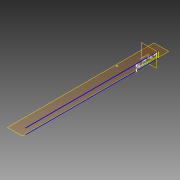
# Autodesk Inventor part: MotorHolder
Saved by Autodesk Inventor 2012 SP2 (Build 160219200, 219)
## iProperties
Created: 2014-02-06
Part Number: MotorHolder
Material: Default
Document SubType Name: Modeling
Designer: 1
Density: 1 g/cm^3
Author: 1
Autodesk Inventor part; units mm, degrees
ref_plane "YZ Plane" through (0, 0, 0) normal (1, 0, 0) x (0, 1, 0)
sketch "Sketch2" plane through (0, 0, 0) normal (1, 0, 0) x (0, 1, 0)
  line L0 (-26.7778, -143.959) -> (-26.7778, 317.1285)
  line L1 (-46.7778, -143.959) -> (-46.7778, 317.1285)
  line L2 (-26.7778, -143.959) -> (-46.7778, -143.959) projected
  line L3 (-39.365, -88.8667) -> (-41.365, -88.8667)
  line L4 (-41.365, -88.8667) -> (-41.365, -138.8667)
  line L5 (-41.365, -138.8667) -> (-39.365, -138.8667)
  line L6 (-39.365, -138.8667) -> (-39.365, -88.8667)
  point P0 (0, 0)
  dimension "d0" = 2
  dimension "d1" = 50
  constraints: 12 end point, 2 parallel, 2 vertical, 1 horizontal, 1 perpendicular, 4 other
  measures "d0" distance of L3.start L3.end
  measures "d1" distance of L3.end L4.end
ref_plane "Work Plane1" through (0, 0, -111.125) normal (0, 0, 1) x (1, 0, 0)
sketch "Sketch3" plane through (0, 0, -111.125) normal (0, 0, 1) x (1, 0, 0)
  line L0 (10, -547.5814) -> (10, 52.4186)
  circle A0 centre (-26.4569, -36.7778) radius 10 projected
  line L1 (-15.1483, -33.3426) -> (-15.1483, -63.4863)
  line L2 (-15.1483, -63.4863) -> (-33.7014, -63.4863)
  point P0 (0, 0)
  constraints: 6 end point, 1 parallel, 1 perpendicular, 1 vertical, 2 other
ref_plane "Work Plane2" through (-15.1483, -33.3426, -111.125) normal (0, 1, 0) x (-1, 0, 0)
sketch "Sketch4" plane through (-15.1483, -33.3426, -111.125) normal (0, 1, 0) x (-1, 0, 0)
  line L0 (1.3086, -144.244) -> (1.3086, 635.626)
  line L1 (1.3086, -32.834) -> (1.3086, 428.2535)
  line L2 (-18.4397, 0) -> (4.6, 0) projected
  line L3 (1.3086, 0) -> (1.3086, -15)
  line L4 (1.3086, -15) -> (-2.1914, -15)
  line L5 (-2.1914, -15) -> (-2.1914, 0)
  line L6 (1.3086, 0) -> (1.3086, 15)
  line L7 (1.3086, 15) -> (-2.1914, 15)
  line L8 (-2.1914, 15) -> (-2.1914, 0)
  point P0 (-15.1483, 111.125)
  dimension "d7" = 15
  dimension "d8" = 3.5
  constraints: 16 end point, 4 point on line, 2 perpendicular, 2 symmetric about line, 2 vertical, 4 other
  measures "d7" distance of L3.start L3.end
  measures "d8" distance of L3.end L4.end
sweep "Sweep1" add profiles "Sketch4" path "Sketch3" path curves L1 L2
fillet "Fillet1" radius 3.5875 1 edges at (-12.9569, -65.6777, -111.125)
fillet "Fillet2" radius 0.4125 1 edges at (-16.4569, -62.1777, -111.125)
sketch "Sketch5" plane through (-33.7014, -62.1777, -96.125) normal (0, 1, 0) x (1, 0, 0)
  line L0 (16.832, 30) -> (16.832, 0) projected
  line L1 (16.832, 30) -> (0, 30) projected
  line L2 (0, 30) -> (0, 0) projected
  line L3 (16.832, 0) -> (0, 0) projected
  line L4 (0, 30) -> (16.832, 0) construction
  line L5 (16.832, 30) -> (0, 0) construction
  line L6 (8.416, 15) -> (16.832, 15) construction
  circle A0 centre (8.416, 15) radius 8.416 construction
  line L7 (16.832, 30) -> (4.03, 22.1828) construction
  line L8 (16.832, 0) -> (4.03, 7.8172) construction
  line L9 (16.832, 30) -> (4.03, 22.1828)
  line L10 (16.832, 0) -> (4.03, 7.8172)
  arc A1 (4.03, 22.1828) -> (4.03, 7.8172) centre (8.416, 15) ccw
  point P0 (33.7014, -96.125)
  constraints: 14 end point, 4 point on circle, 4 tangent, 2 centre point, 2 coincident, 2 collinear, 2 midpoint
extrude "Extrusion1" cut sketch "Sketch5" against normal blind 10 contours L9 A1 L2 L1 | L3 L2 A1 L10
sketch "Sketch6" plane through (-16.8694, -62.1777, -96.125) normal (0, 1, 0) x (1, 0, 0)
  arc A0 (-12.802, 22.1828) -> (-12.802, 7.8172) centre (-8.416, 15) ccw projected
  circle A1 centre (-8.416, 15) radius 4.386
  point P0 (16.8694, -96.125)
  constraints: 1 centre point, 1 coincident
extrude "Extrusion2" cut sketch "Sketch6" against normal through all
sketch "Sketch7" plane through (-16.4569, -33.3426, -96.125) normal (0, 1, 0) x (1, 0, 0)
  line L0 (0, 30) -> (0, 0) projected
  line L1 (0, 0) -> (3.5, 0) projected
  line L2 (3.5, 0) -> (3.5, 30) projected
  line L3 (3.5, 30) -> (0, 30) projected
  point P0 (16.4569, -96.125)
extrude "Extrusion3" add sketch "Sketch7" along normal blind 8.4125
body "Solid1"
